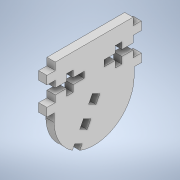
# Autodesk Inventor part: crashy
Saved by Autodesk Inventor 2020 (Build 240168000, 168)
## iProperties
Created: 2019-07-10
Material: Générique
Document SubType Name: Modeling
Designer: Thibault
Density: 1 g/cm^3
Appearance: Par défaut
angle: 27.00 deg
Author: Thibault
Autodesk Inventor part; units mm, degrees
ref_plane "YZ Plane" through (0, 0, 0) normal (1, 0, 0) x (0, 1, 0)
ref_plane "XZ Plane" through (0, 0, 0) normal (0, 1, 0) x (-1, 0, 0)
ref_plane "XY Plane" through (0, 0, 0) normal (0, 0, 1) x (1, 0, 0)
sketch "Half" plane through (0, 0, 0) normal (0, 0, 1) x (1, 0, 0)
  line L0 (20, 19.8752) -> (18.6728, 19.8752)
  line L1 (18.6728, 19.8752) -> (18.6728, 21.3752)
  line L2 (18.6728, 21.3752) -> (17.1728, 21.3752)
  line L3 (17.1728, 21.3752) -> (17.1728, 19.8752)
  line L4 (13.6728, 19.8752) -> (13.6728, 21.3752)
  line L5 (13.6728, 21.3752) -> (12.1728, 21.3752)
  line L6 (12.1728, 21.3752) -> (12.1728, 20.0756)
  line L7 (20, 19.8752) -> (20, 12.8752)
  line L8 (17.1728, 19.8752) -> (15.9728, 19.8752)
  line L9 (15.9728, 19.8752) -> (15.9728, 17.8752)
  line L10 (15.9728, 17.8752) -> (17.1728, 17.8752)
  line L11 (17.1728, 17.8752) -> (17.1728, 16.6752)
  line L12 (17.1728, 16.6752) -> (15.9728, 16.6752)
  line L13 (15.9728, 16.6752) -> (15.9728, 14.6752)
  line L14 (15.9728, 14.6752) -> (14.8728, 14.6752)
  line L15 (14.8728, 14.6752) -> (14.8728, 16.6752)
  line L16 (14.8728, 16.6752) -> (13.6728, 16.6752)
  line L17 (13.6728, 16.6752) -> (13.6728, 17.8752)
  line L18 (13.6728, 17.8752) -> (14.8728, 17.8752)
  line L19 (14.8728, 17.8752) -> (14.8728, 19.8752)
  line L20 (14.8728, 19.8752) -> (13.6728, 19.8752)
  line L21 (21, 12.8752) -> (-1, 12.8752) construction
  line L22 (12.1728, 20.0756) -> (10.6728, 20.0756)
  arc A0 (10.6728, 20.0756) -> (3.5349, 12.8752) centre (10.7356, 12.8752) ccw
  point P0 (14.6929, 17.8988)
  dimension "d0" = 1.5
  dimension "d1" = 1.5
  dimension "d2" = 3.5
  dimension "d3" = 7
  dimension "d4" = 1.5
  dimension "d6" = 2
  dimension "d7" = 1.2
  dimension "d8" = 1.2
  dimension "d10" = 2
  dimension "d11" = 1.1
  dimension "d12" = 1.2
  dimension "d13" = 1.5
  measures "d0" distance of L0.end L1.end
  measures "d1" distance of L1.end L2.end
  measures "d2" distance of L3.end L4.start
  measures "d3" distance of L0.start L7.end
  measures "d4" distance of L4.end L5.end
  measures "d6" distance of L8.end L9.end
  measures "d7" distance of L9.end L10.end
  measures "d8" distance of L10.end L11.end
  measures "d10" distance of L12.end L14.start
  measures "d11" distance of L14.start L14.end
  measures "d12" distance of L15.end L16.end
  measures "d13" distance of L6.end L22.end
sketch "Esquisse1" plane through (0, 0, 0) normal (1, 0, 0) x (0, 1, 0)
  line L0 (21.693, 16.703) -> (20.3565, 17.384)
  line L1 (20.3565, 17.384) -> (19.6755, 16.0475)
  line L2 (19.6755, 16.0475) -> (21.012, 15.3665)
  line L3 (21.012, 15.3665) -> (21.693, 16.703)
  line L4 (21.693, 16.703) -> (19.6755, 16.0475) construction
  line L5 (20.3565, 17.384) -> (21.012, 15.3665) construction
  line L6 (20.6843, 16.3752) -> (1.0186, 26.3954)
  line L7 (17.238, 18.9729) -> (16.557, 17.6364)
  line L8 (16.557, 17.6364) -> (17.8935, 16.9554)
  line L9 (17.8935, 16.9554) -> (18.5745, 18.292)
  line L10 (18.5745, 18.292) -> (17.238, 18.9729)
  line L11 (17.238, 18.9729) -> (17.8935, 16.9554) construction
  line L12 (16.557, 17.6364) -> (18.5745, 18.292) construction
  line L13 (13.4385, 19.2254) -> (14.775, 18.5444)
  line L14 (14.775, 18.5444) -> (15.456, 19.8809)
  line L15 (15.456, 19.8809) -> (14.1195, 20.5619)
  line L16 (14.1195, 20.5619) -> (14.775, 18.5444) construction
  line L17 (13.4385, 19.2254) -> (15.456, 19.8809) construction
  line L18 (29.9487, 23.3752) -> (28.6215, 23.3752)
  line L19 (28.6215, 23.3752) -> (28.6215, 24.8752)
  line L20 (28.6215, 24.8752) -> (27.1215, 24.8752)
  line L21 (27.1215, 24.8752) -> (27.1215, 23.3752)
  line L22 (23.6215, 23.3752) -> (23.6215, 24.8752)
  line L23 (23.6215, 24.8752) -> (22.1215, 24.8752)
  line L24 (22.1215, 24.8752) -> (22.1215, 23.5756)
  line L25 (29.9487, 23.3752) -> (29.9487, 16.3752)
  line L26 (27.1215, 23.3752) -> (25.9215, 23.3752)
  line L27 (25.9215, 23.3752) -> (25.9215, 21.3752)
  line L28 (25.9215, 21.3752) -> (27.1215, 21.3752)
  line L29 (27.1215, 21.3752) -> (27.1215, 20.1752)
  line L30 (27.1215, 20.1752) -> (25.9215, 20.1752)
  line L31 (25.9215, 20.1752) -> (25.9215, 18.1752)
  line L32 (25.9215, 18.1752) -> (24.8215, 18.1752)
  line L33 (24.8215, 18.1752) -> (24.8215, 20.1752)
  line L34 (24.8215, 20.1752) -> (23.6215, 20.1752)
  line L35 (23.6215, 20.1752) -> (23.6215, 21.3752)
  line L36 (23.6215, 21.3752) -> (24.8215, 21.3752)
  line L37 (24.8215, 21.3752) -> (24.8215, 23.3752)
  line L38 (24.8215, 23.3752) -> (23.6215, 23.3752)
  line L39 (30.9487, 16.3752) -> (8.9487, 16.3752) construction
  line L40 (22.1215, 23.5756) -> (20.6215, 23.5756)
  arc A0 (20.6215, 23.5756) -> (13.4836, 16.3752) centre (20.6843, 16.3752) ccw
  line L41 (29.9487, 9.3752) -> (28.6215, 9.3752)
  line L42 (28.6215, 9.3752) -> (28.6215, 7.8752)
  line L43 (28.6215, 7.8752) -> (27.1215, 7.8752)
  line L44 (27.1215, 7.8752) -> (27.1215, 9.3752)
  line L45 (23.6215, 9.3752) -> (23.6215, 7.8752)
  line L46 (23.6215, 7.8752) -> (22.1215, 7.8752)
  line L47 (22.1215, 7.8752) -> (22.1215, 9.1749)
  line L48 (29.9487, 9.3752) -> (29.9487, 16.3752)
  line L49 (27.1215, 9.3752) -> (25.9215, 9.3752)
  line L50 (25.9215, 9.3752) -> (25.9215, 11.3752)
  line L51 (25.9215, 11.3752) -> (27.1215, 11.3752)
  line L52 (27.1215, 11.3752) -> (27.1215, 12.5752)
  line L53 (27.1215, 12.5752) -> (25.9215, 12.5752)
  line L54 (25.9215, 12.5752) -> (25.9215, 14.5752)
  line L55 (25.9215, 14.5752) -> (24.8215, 14.5752)
  line L56 (24.8215, 14.5752) -> (24.8215, 12.5752)
  line L57 (24.8215, 12.5752) -> (23.6215, 12.5752)
  line L58 (23.6215, 12.5752) -> (23.6215, 11.3752)
  line L59 (23.6215, 11.3752) -> (24.8215, 11.3752)
  line L60 (24.8215, 11.3752) -> (24.8215, 9.3752)
  line L61 (24.8215, 9.3752) -> (23.6215, 9.3752)
  line L62 (30.9487, 16.3752) -> (8.9487, 16.3752) construction
  line L63 (22.1215, 9.1749) -> (20.6215, 9.1749)
  arc A1 (20.6215, 9.1749) -> (13.4836, 16.3752) centre (20.6843, 16.3752) cw
  point P0 (0, 0)
  point P1 (20.6843, 16.3752)
  point P2 (13.6851, 23.3744)
  point P3 (13.6851, 23.3744)
  point P4 (17.5658, 17.9642)
  point P5 (17.5658, 17.9642)
  point P6 (14.4472, 19.5532)
  point P7 (14.4472, 19.5532)
  point P8 (13.9629, 18.9582)
  point P9 (14.6439, 20.2947)
  dimension "d16" = 1.5
  dimension "d17" = 1.5
  dimension "d21" = 1.5
  dimension "d22" = 1.5
  dimension "d24" = 2
  dimension "d26" = 1.5
  dimension "d27" = 1.5
  dimension "d28" = 2
  constraints: 36 end point, 9 midpoint, 8 parallel, 2 perpendicular, 2 point on line, 2 other
  measures "d16" distance of L2.end L1.end
  measures "d17" distance of L1.end L0.end
  measures "d21" distance of L9.end L8.end
  measures "d22" distance of L8.end L7.end
  measures "d24" distance of L0.end L9.end
  measures "d26" distance of L14.end L13.end
  measures "d27" distance of L13.end L13.start
  measures "d28" distance between parallel lines of L14 L7
extrude "Extrusion1" add sketch "Esquisse1" along normal blind 1.5 contours L14 L15 A0 L40 L24 L23 L22 L38 L37 L36 L35 L34 L33 L32 L31 L30 L29 L28 L27 L26 L21 L20 L19 L18 L25 L48 L41 L42 L43 L44 L49 L50 L51 L52 L53 L54 L55 L56 L57 L58 L59 L60 L61 L45 L46 L47 L63 A1 L13
equation "\"d7\" = d12"
equation "\"d10\" = d6"
